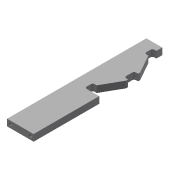
# Autodesk Inventor part: Olfactometer_Holder
Saved by Autodesk Inventor 2016 (Build 200138000, 138)
## iProperties
Created: 2013-03-04
Part Number: Olfactometer_Holder
Material: Stainless Steel
Document SubType Name: Modeling
Designer: Neef
Density: 8 g/cm^3
Appearance: Semi-Polished
Author: Neef
Autodesk Inventor part; units mm, degrees
ref_plane "YZ Plane" through (0, 0, 0) normal (1, 0, 0) x (0, 1, 0)
ref_plane "XZ Plane" through (0, 0, 0) normal (0, 1, 0) x (-1, 0, 0)
ref_plane "XY Plane" through (0, 0, 0) normal (0, 0, 1) x (1, 0, 0)
sketch "Skizze1" plane through (0, 0, 0) normal (0, 0, 1) x (1, 0, 0)
  line L0 (0, 42) -> (0, -252) projected
  line L1 (-28, 0) -> (28, 0) projected
  line L2 (20, 0) -> (-20, 0)
  line L3 (-20, 0) -> (-20, -210)
  line L4 (-20, -210) -> (20, -210)
  line L5 (20, -210) -> (20, 0)
  point P0 (0, 0)
  point P1 (0, -210)
  dimension "d0" = 210
  dimension "d1" = 40
  constraints: 8 end point, 2 parallel, 1 collinear, 1 horizontal, 1 midpoint, 1 perpendicular, 1 point on line
  measures "d0" distance of L4.end L2.start
  measures "d1" distance of L3.end L4.end
extrude "Extrusion1" add sketch "Skizze1" along normal blind 10
sketch "Skizze2" plane through (0, 0, 10) normal (0, 0, 1) x (1, 0, 0)
  line L0 (20, 0) -> (20, -210) projected
  line L1 (-20, 0) -> (20, 0) projected
  line L2 (20, -8.9) -> (1, -8.9)
  line L3 (-2, -11.9) -> (-2, -18.1)
  line L4 (1, -21.1) -> (20, -21.1)
  line L5 (20, -21.1) -> (20, -8.9)
  arc A0 (1, -8.9) -> (-2, -11.9) centre (1, -11.9) ccw
  arc A1 (-2, -18.1) -> (1, -21.1) centre (1, -18.1) ccw
  line L6 (1, -12) -> (1, -18) construction
  line L7 (20, -52.4) -> (17, -52.4)
  line L8 (14, -55.4) -> (14, -64.6)
  line L9 (17, -67.6) -> (20, -67.6)
  line L10 (20, -67.6) -> (20, -52.4)
  arc A2 (17, -52.4) -> (14, -55.4) centre (17, -55.4) ccw
  arc A3 (14, -64.6) -> (17, -67.6) centre (17, -64.6) ccw
  line L11 (17, -55.5) -> (17, -64.5) construction
  line L12 (20, -98.9) -> (1, -98.9)
  line L13 (-2, -101.9) -> (-2, -108.1)
  line L14 (1, -111.1) -> (20, -111.1)
  line L15 (20, -111.1) -> (20, -98.9)
  arc A4 (1, -98.9) -> (-2, -101.9) centre (1, -101.9) ccw
  arc A5 (-2, -108.1) -> (1, -111.1) centre (1, -108.1) ccw
  line L16 (1, -102) -> (1, -108) construction
  point P0 (0, 0)
  dimension "d4" = 22
  dimension "d5" = 12.2
  dimension "d6" = 3
  dimension "d7" = 6
  dimension "d8" = 0.1
  dimension "d9" = 12
  dimension "d10" = 6
  dimension "d11" = 15.2
  dimension "d12" = 3
  dimension "d13" = 9
  dimension "d14" = 0.1
  dimension "d15" = 55.5
  dimension "d16" = 12.2
  dimension "d17" = 22
  dimension "d18" = 3
  dimension "d19" = 6
  dimension "d20" = 0.1
  dimension "d21" = 102
  constraints: 30 end point, 12 point on circle, 12 tangent, 9 parallel, 6 centre point, 6 point on line, 3 equal radius, 3 horizontal, 3 perpendicular
  measures "d4" distance between parallel lines of L5 L3
  measures "d5" distance between parallel lines of L4 L2
  measures "d6" radius of A0
  measures "d7" distance of L6.start L6.end
  measures "d8" distance of A1.centre L6.end
  measures "d9" distance from line of L1 L6.start
  measures "d10" distance between parallel lines of L0 L8
  measures "d11" distance between parallel lines of L9 L7
  measures "d12" radius of A2
  measures "d13" distance of L11.start L11.end
  measures "d14" distance of A3.centre L11.end
  measures "d15" distance from line of L1 L11.start
  measures "d16" distance between parallel lines of L14 L12
  measures "d17" distance between parallel lines of L0 L13
  measures "d18" radius of A4
  measures "d19" distance of L16.start L16.end
  measures "d20" distance of A5.centre L16.end
  measures "d21" distance from line of L1 L16.start
extrude "Extrusion2" cut sketch "Skizze2" against normal through all
sketch "Skizze3" plane through (0, 0, 0) normal (0, 0, -1) x (-1, 0, 0)
  line L0 (-20, -98.9) -> (-1, -98.9) projected
  line L1 (-20, 0) -> (20, 0) projected
  line L2 (-20, -8.9) -> (-20, 0) projected
  line L3 (-20, -8.9) -> (-1, -8.9) projected
  line L4 (-1, -21.1) -> (-20, -21.1) projected
  line L5 (-20, -52.4) -> (-20, -21.1) projected
  line L6 (-20, -52.4) -> (-17, -52.4) projected
  line L7 (-17, -67.6) -> (-20, -67.6) projected
  line L8 (-20, -98.9) -> (-20, -67.6) projected
  line L9 (-20, -49.4) -> (-4, -21.1)
  line L10 (-4, -8.9) -> (-4, 0)
  line L11 (-20, -70.6) -> (-4, -98.9)
  point P0 (0, 0)
  dimension "d24" = 3
  dimension "d25" = 3
  dimension "d26" = 16
  dimension "d27" = 3
  dimension "d28" = 3
  constraints: 6 end point, 6 point on line, 1 perpendicular
  measures "d24" distance from line of L9.start L6
  measures "d25" distance of L4.start L9.end
  measures "d26" distance between parallel lines of L2 L10
  measures "d27" distance of L0.end L11.end
  measures "d28" distance from line of L7 L11.start
extrude "Extrusion3" cut sketch "Skizze3" against normal through all
sketch "Skizze4" plane through (-20, -210, 0) normal (0, -1, 0) x (1, 0, 0)
  line L0 (0, 0) -> (40, 0) projected
  line L1 (40, 0) -> (40, 10) projected
  point P0 (20, 0)
  point P1 (5, 5)
  point P2 (35, 5)
  dimension "d31" = 30
  dimension "d32" = 5
  dimension "d33" = 5
  dimension "d34" = 5
  measures "d31" distance of point (35, 5) point (5, 5)
  measures "d32" distance from line of L1 point (35, 5)
  measures "d33" distance from line of L0 point (35, 5)
  measures "d34" distance from line of point (5, 5) L0
hole "Bohrung1" at (-15, -210, 5) at (15, -210, 5) direction (0, 1, 0) diameter 4.134 depth 15 tip angle 118 thread size "M5x0.8" class "6H" standard "ISO Metric profile"
equation "\"d16\" = d5"
equation "\"d17\" = d4"
equation "\"d18\" = d6"
equation "\"d27\" = d25"
equation "\"d28\" = d24"
equation "\"d34\" = d33"
